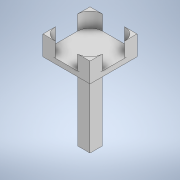
# Autodesk Inventor part: CenterClawv2.2
Saved by Autodesk Inventor 2021 (Build 250183000, 183)
## iProperties
Created: 2024-01-12
Part Number: CenterClawv2.2
Material: Generic
Document SubType Name: Modeling
Designer: brybr
Density: 1 g/cm^3
Appearance: Default
Author: brybr
Autodesk Inventor part; units mm, degrees
ref_plane "YZ Plane" through (0, 0, 0) normal (1, 0, 0) x (0, 1, 0)
ref_plane "XZ Plane" through (0, 0, 0) normal (0, 1, 0) x (-1, 0, 0)
ref_plane "XY Plane" through (0, 0, 0) normal (0, 0, 1) x (1, 0, 0)
sketch "Sketch1" plane through (0, 0, 0) normal (0, 1, 0) x (-1, 0, 0)
  line L0 (-9.5, 9.5) -> (9.5, 9.5)
  line L1 (9.5, 9.5) -> (9.5, -9.5)
  line L2 (9.5, -9.5) -> (-9.5, -9.5)
  line L3 (-9.5, -9.5) -> (-9.5, 9.5)
  line L4 (-9.5, 9.5) -> (9.5, -9.5) construction
  line L5 (9.5, 9.5) -> (-9.5, -9.5) construction
  line L6 (9.5, 0) -> (9.5, 4.5)
  line L7 (9.5, 0) -> (14, 0) construction
  line L8 (0, 9.5) -> (4.5, 9.5)
  line L9 (0, 9.5) -> (4.5, 9.5) construction
  arc A0 (9.5, 4.5) -> (4.5, 9.5) centre (4.5, 4.5) ccw
  arc A1 (-4.5, 9.5) -> (-9.5, 4.5) centre (-4.5, 4.5) ccw
  arc A2 (-9.5, -4.5) -> (-4.5, -9.5) centre (-4.5, -4.5) ccw
  arc A3 (4.5, -9.5) -> (9.5, -4.5) centre (4.5, -4.5) ccw
  point P0 (0, 0)
  point P1 (9.5, -4.5)
  point P2 (-4.5, 9.5)
  point P3 (-9.5, 4.5)
  point P4 (-9.5, -4.5)
  point P5 (-4.5, -9.5)
  dimension "d0" = 19
  dimension "d1" = 19
  dimension "d2" = 4.5
  dimension "d3" = 90
  dimension "d4" = 4.5
  dimension "d5" = 0
  dimension "d6" = 5
  dimension "d9" = 360
  constraints: 20 end point, 8 point on circle, 4 centre point, 4 midpoint, 3 horizontal, 2 collinear, 2 equal length, 2 parallel, 1 perpendicular, 17 other
  measures "d0" distance of L1.end L2.end
  measures "d1" distance of L0.end L1.end
  measures "d2" distance of L6.start L6.end
  measures "d3" angle of L7 L6
  measures "d4" distance of L8.start L8.end
  measures "d5" distance between parallel lines of L8 L9
  measures "d6" radius of A0
extrude "Extrusion1" add sketch "Sketch1" along normal blind 2 contours L0 A0 L1 A3 L2 A2 L3 A1
extrude "Extrusion2" add sketch "Sketch1" along normal blind 8 contours L0 A1 L3 | A2 L2 L3 | L0 L1 A0 | A3 L1 L2
sketch "Sketch2" plane through (0, 0, 0) normal (0, -1, 0) x (1, 0, 0)
  line L0 (-2.45, 2.45) -> (-2.45, -2.45)
  line L1 (-2.45, -2.45) -> (2.45, -2.45)
  line L2 (2.45, -2.45) -> (2.45, 2.45)
  line L3 (2.45, 2.45) -> (-2.45, 2.45)
  line L4 (-2.45, 2.45) -> (2.45, -2.45) construction
  line L5 (-2.45, -2.45) -> (2.45, 2.45) construction
  line L6 (-2.45, 2.45) -> (2.45, 2.45) construction
  point P0 (0, 0)
  dimension "d22" = 4.9
  dimension "d23" = 90
  dimension "d24" = 4.9
  constraints: 14 end point, 2 midpoint, 2 parallel, 2 perpendicular, 1 horizontal, 1 vertical
  measures "d22" distance of L0.start L0.end
  measures "d23" angle of L0 L6
  measures "d24" distance of L1.end L0.end
extrude "Extrusion3" add sketch "Sketch2" along normal blind 31.25
body "Solid1"
